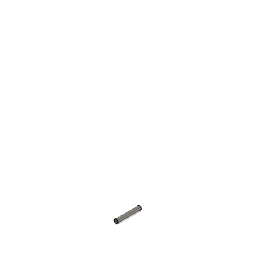
splicer_camera_rgb-filter_axle (Autodesk Fusion 360 design; units mm, degrees)
Autodesk Fusion 360 part; units mm, degrees
sketch "Sketch1" plane through (0, 0, -188.6) normal (0, 0, -1) x (0.707107, -0.707107, 0)
  circle A0 centre (46.0559, 45.8678) radius 6.65
  circle A1 centre (46.0559, 45.8678) radius 2.475
  dimension "d167" = 4.95
  constraint concentric A0 A1
  measures "d167" diameter of A1
extrude "Extrude1" add sketch "Sketch1" along normal blind 30 contours A1
named bodies: "splicer_camera_rgb-filter_axle"
